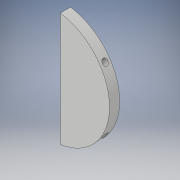
# Autodesk Inventor part: ContrapesoGrande
Saved by Autodesk Inventor 2019 (Build 230136000, 136)
## iProperties
Created: 2019-06-29
Part Number: ContrapesoGrande
Material: Generic
Document SubType Name: Modeling
Designer: usuario
Density: 1 g/cm^3
Appearance: Default
Mass: 16.5969 g
Surface Area: 68.3967 cm^2
Volume: 16.5969 cm^3
Author: usuario
Autodesk Inventor part; units mm, degrees
ref_plane "YZ Plane" through (0, 0, 0) normal (1, 0, 0) x (0, 1, 0)
ref_plane "XZ Plane" through (0, 0, 0) normal (0, 1, 0) x (-1, 0, 0)
ref_plane "XY Plane" through (0, 0, 0) normal (0, 0, 1) x (1, 0, 0)
sketch "Sketch3" plane through (0, 0, 0) normal (0, 0, 1) x (1, 0, 0)
  arc A0 (6.2115, -31.9009) -> (6.2115, 31.9009) centre (0, 0) ccw
  line L0 (6.2115, 27.4733) -> (6.2115, 31.9009)
  line L1 (6.2115, 31.9009) -> (6.2115, -31.9009)
  circle A1 centre (0, 0) radius 42.5
  line L2 (6.2115, -31.9009) -> (6.2115, -42.0436)
  line L3 (6.2115, 31.9009) -> (6.2115, 42.0436)
  point P0 (-5.2115, 24.6247)
  dimension "d14" = 85
  constraints: 8 end point, 4 point on circle, 2 centre point, 2 coincident, 2 vertical, 1 point on line
  measures "d14" diameter of A1
extrude "Extrusion2" add sketch "Sketch3" along normal blind 7.5 contours L1 L0 A0
sketch "Sketch4" plane through (6.2115, -31.9009, 0) normal (-1, 0, 0) x (0, 0, 1)
  line L0 (0, 0) -> (0, 6.9167)
  line L1 (7.5, 26.7893) -> (7.5, 0)
  line L2 (7.5, 6.9167) -> (7.5, 0)
  line L3 (7.5, 0) -> (0, 0)
  line L4 (7.5, 0) -> (0, 0)
  circle A0 centre (3.75, 8.5699) radius 1
  line L5 (0, 0) -> (3.0149, 2.7804)
  line L6 (4.4851, 4.1363) -> (7.5, 6.9167)
  line L7 (0, 6.9167) -> (3.0149, 4.1363)
  line L8 (4.4851, 2.7804) -> (7.5, 0)
  line L9 (0, 0) -> (0, 53.5786)
  line L10 (0, 53.5786) -> (0, 0)
  line L11 (0, 31.9009) -> (7.5, 31.9009)
  circle A1 centre (3.75, 55.2319) radius 1
  line L12 (7.5, 53.5786) -> (7.5, 0)
  line L13 (0, 0) -> (0, 63.8018) projected
  line L14 (0, 63.8018) -> (0, 0)
  line L15 (0, 31.9009) -> (3.75, 31.9009)
  circle A2 centre (3.75, 8.5699) radius 2
  circle A3 centre (3.75, 55.2319) radius 2
  point P0 (280.32, 51.414)
  dimension "d7" = 2
  dimension "d10" = 4
  dimension "d11" = 4
  constraints: 30 end point, 4 centre point, 3 collinear, 2 coincident, 2 vertical, 1 horizontal, 1 perpendicular, 1 symmetric about line, 1 other
  measures "d7" diameter of A0
  measures "d10" diameter of A2
  measures "d11" diameter of A3
extrude "Extrusion3" cut sketch "Sketch4" against normal blind 25.4 contours A0 | A1
extrude "Extrusion4" cut sketch "Sketch4" against normal blind 32.8625 contours A2 | A3
extrude "Extrusion5" add sketch "Sketch3" along normal blind 7.5 contours A0 L3 A1 L2
extrude "Extrusion6" cut sketch "Sketch4" against normal blind 50.3625 contours A0 | A1 | A2 | A3
body "Solid2"
